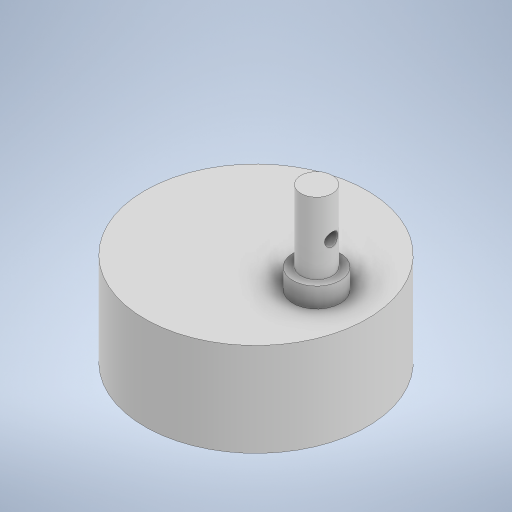
# Autodesk Inventor part: 24W_motor
Saved by Autodesk Inventor 2023 (Build 270158000, 158)
## iProperties
Created: 2026-05-06
Part Number: 24W_motor
Material: Generic
Document SubType Name: Modeling
Designer: Justin Pascual
Density: 1 g/cm^3
Appearance: Default
Author: Justin Pascual
Autodesk Inventor part; units mm, degrees
ref_plane "YZ Plane" through (0, 0, 0) normal (1, 0, 0) x (0, 1, 0)
ref_plane "XZ Plane" through (0, 0, 0) normal (0, 1, 0) x (-1, 0, 0)
ref_plane "XY Plane" through (0, 0, 0) normal (0, 0, 1) x (1, 0, 0)
sketch "Sketch1" plane through (0, 0, 0) normal (0, 1, 0) x (-1, 0, 0)
  circle A0 centre (0, 0) radius 24.638
  dimension "d0" = 49.276
  constraints: 1 centre point, 1 coincident
  measures "d0" diameter of A0
extrude "Extrusion1" add sketch "Sketch1" along normal blind 20.701
sketch "Sketch2" plane through (0, 20.701, 0) normal (0, 1, 0) x (1, 0, 0)
  circle A0 centre (13.4366, 0) radius 3.4925
  point P0 (0, 0)
  dimension "d3" = 6.985
  dimension "d4" = 13.4366
  constraints: 1 centre point
  measures "d3" diameter of A0
  measures "d4" distance of A0.centre point (0, 0)
extrude "Extrusion2" add sketch "Sketch2" along normal blind 20.2184
sketch "Sketch3" plane through (0, 20.701, 0) normal (0, 1, 0) x (1, 0, 0)
  circle A0 centre (13.4366, 0) radius 3.4925 projected
  circle A1 centre (13.4366, 0) radius 5.2451
  point P0 (0, 0)
  dimension "d7" = 10.4902
  constraints: 1 centre point, 1 coincident
  measures "d7" diameter of A1
extrude "Extrusion3" add sketch "Sketch3" along normal blind 4.3942 contours A0 | A1
sketch "Sketch4" plane through (0, 0, 0) normal (1, 0, 0) x (0, 1, 0)
  circle A0 centre (32.131, 0) radius 1.4605
  line L0 (20.701, -24.638) -> (20.701, 24.638) projected
  point P0 (0, 0)
  dimension "d10" = 2.921
  dimension "d11" = 11.43
  constraints: 1 centre point
  measures "d10" diameter of A0
  measures "d11" distance from line of L0 A0.centre
extrude "Extrusion4" cut sketch "Sketch4" along normal through all
body "Solid1"
